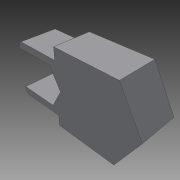
# Autodesk Inventor part: nut_tool
Saved by Autodesk Inventor 2014 (Build 180170000, 170)
## iProperties
Created: 2014-04-22
Part Number: nut_tool
Material: Plywood, Finish
Document SubType Name: Modeling
Designer: buben
Density: 0.552 g/cm^3
Appearance: Plywood - New
Author: buben
Autodesk Inventor part; units mm, degrees
ref_plane "YZ Plane" through (0, 0, 0) normal (1, 0, 0) x (0, 1, 0)
ref_plane "XZ Plane" through (0, 0, 0) normal (0, 1, 0) x (-1, 0, 0)
ref_plane "XY Plane" through (0, 0, 0) normal (0, 0, 1) x (1, 0, 0)
sketch "Sketch1" plane through (0, 0, 0) normal (0, 1, 0) x (-1, 0, 0)
  line L0 (-2.0207, 3.5) -> (5, 3.5)
  line L1 (5, -3.5) -> (-2.0207, -3.5)
  line L2 (-2.0207, -3.5) -> (-4.0415, 0)
  line L3 (-4.0415, 0) -> (-2.0207, 3.5)
  line L4 (5, -3.5) -> (5, -4.75)
  line L5 (5, -4.75) -> (-3.25, -4.75)
  line L6 (5, 3.5) -> (5, 4.75)
  line L7 (5, 4.75) -> (-3.25, 4.75)
  line L8 (-3.25, -4.75) -> (-3.25, -6.75)
  line L9 (-3.25, 4.75) -> (-3.25, 6.75)
  line L10 (-3.25, -6.75) -> (-14.3529, -6.75)
  line L11 (-14.3529, -6.75) -> (-18.25, 0)
  line L12 (-18.25, 0) -> (-14.3529, 6.75)
  line L13 (-3.25, 6.75) -> (-14.3529, 6.75)
  point P0 (0, 0)
  point P1 (0, 0)
  dimension "d1" = 7
  dimension "d2" = 9.5
  dimension "d3" = 5
  dimension "d4" = 3.25
  dimension "d5" = 15
  dimension "d6" = 2
  constraints: 28 end point, 7 perpendicular, 5 collinear, 3 parallel, 1 coincident, 1 horizontal, 1 horizontal alignment, 6 other
  measures "d1" distance between parallel lines of L1 L0
  measures "d2" distance between parallel lines of L7 L5
  measures "d3" distance from line of point (0, 0) L6
  measures "d4" distance from line of point (0, 0) L8
  measures "d5" distance from line of L11.end L9
  measures "d6" distance of L7.end L9.end
extrude "Extrusion1" add sketch "Sketch1" along normal blind 6.5
chamfer "Chamfer1" distance 0.5 angle 45 2 edges at (-5, 3.25, -4.75) (-5, 3.25, 4.75)
body "Solid1"
